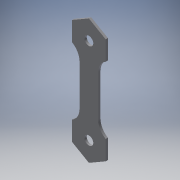
# Autodesk Inventor part: Leg
Saved by Autodesk Inventor 2016 (Build 200138000, 138)
## iProperties
Created: 2015-10-16
Part Number: Leg
Material: Generic
Document SubType Name: Modeling
Designer: powasar16
Density: 1 g/cm^3
Appearance: Default
Author: powasar16
Autodesk Inventor part; units mm, degrees
ref_plane "YZ Plane" through (0, 0, 0) normal (1, 0, 0) x (0, 1, 0)
ref_plane "XZ Plane" through (0, 0, 0) normal (0, 1, 0) x (-1, 0, 0)
ref_plane "XY Plane" through (0, 0, 0) normal (0, 0, 1) x (1, 0, 0)
sketch "Sketch1" plane through (0, 0, 0) normal (0, 0, 1) x (1, 0, 0)
  circle A0 centre (2.8854, -1.4956) radius 3.75 projected
  line L0 (2.8854, 15.0022) -> (17.1729, 6.7533)
  line L1 (17.1729, 6.7533) -> (17.1729, -9.7445)
  line L2 (17.1729, -9.7445) -> (2.8854, -17.9934) construction
  line L3 (2.8854, -17.9934) -> (-11.4021, -9.7445) construction
  line L4 (-11.4021, -9.7445) -> (-11.4021, 6.7533)
  line L5 (-11.4021, 6.7533) -> (2.8854, 15.0022)
  line L6 (-5.0521, -13.4107) -> (10.8229, -13.4107) construction
  line L7 (10.8229, -13.4107) -> (10.8229, -20.743) construction
  line L8 (10.8229, -59.433) -> (-5.0521, -59.433) construction
  line L9 (-5.0521, -59.433) -> (-5.0521, -52.0982) construction
  line L10 (10.8229, -36.4206) -> (-5.0521, -36.4206) construction
  arc A1 (17.1729, -9.7445) -> (10.8229, -20.743) centre (23.5229, -20.743) ccw
  line L11 (2.8854, -13.4107) -> (2.8854, -59.433) construction
  arc A2 (-5.0521, -20.743) -> (-11.4021, -9.7445) centre (-17.7521, -20.743) ccw
  circle A3 centre (2.8854, -71.3456) radius 3.75
  line L12 (2.8854, -87.8434) -> (17.1729, -79.5945)
  line L13 (17.1729, -79.5945) -> (17.1729, -63.0967)
  line L14 (17.1729, -63.0967) -> (2.8854, -54.8478) construction
  line L15 (2.8854, -54.8478) -> (-11.4021, -63.0967) construction
  line L16 (-11.4021, -63.0967) -> (-11.4021, -79.5945)
  line L17 (-11.4021, -79.5945) -> (2.8854, -87.8434)
  arc A4 (10.8229, -52.0982) -> (17.1729, -63.0967) centre (23.5229, -52.0982) ccw
  arc A5 (-11.4021, -63.0967) -> (-5.0521, -52.0982) centre (-17.7521, -52.0982) ccw
  line L18 (10.8229, -20.743) -> (10.8229, -52.0982)
  line L19 (-5.0521, -20.743) -> (-5.0521, -13.4107) construction
  line L20 (-5.0521, -52.0982) -> (-5.0521, -20.743)
  line L21 (10.8229, -52.0982) -> (10.8229, -59.433) construction
  point P0 (0, 0)
  dimension "d2" = 28.575
  dimension "d3" = 15.875
  dimension "d6" = 34.925
  dimension "d7" = 11.9151
  dimension "d8" = 11.9126
  constraints: 44 end point, 13 symmetric about line, 10 parallel, 8 point on circle, 4 centre point, 4 tangent, 3 perpendicular, 2 midpoint, 2 point on line, 1 coincident, 1 horizontal, 17 other
  measures "d2" distance between parallel lines of L1 L4
  measures "d3" distance between parallel lines of L7 L9
  measures "d6" distance from line of A0.centre L10
  measures "d7" distance from line of A0.centre L6
  measures "d8" distance from line of L8 A3.centre
extrude "Extrusion1" add sketch "Sketch1" along normal blind 1.905
body "Solid1"
